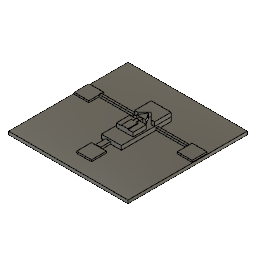
fixture v5 (Autodesk Fusion 360 design; units mm, degrees)
Autodesk Fusion 360 part; units mm, degrees
sketch "base plate" plane through (0, 0, 0) normal (0, 0, 1) x (1, 0, 0)
  line L0 (-228.6, 228.6) -> (228.6, 228.6)
  line L1 (228.6, 228.6) -> (228.6, -228.6)
  line L2 (228.6, -228.6) -> (-228.6, -228.6)
  line L3 (-228.6, -228.6) -> (-228.6, 228.6)
  line L4 (-228.6, 228.6) -> (228.6, -228.6) construction
  line L5 (228.6, 228.6) -> (-228.6, -228.6) construction
  dimension "d1" = 457.2
  dimension "d2" = 457.2
  constraint horizontal L0
  constraint perpendicular L0 L1
  constraint parallel L0 L2
  constraint parallel L1 L3
  constraint coincident L4 origin
  constraint coincident L5 origin
  measures "d1" distance of L1.end L2.end
  measures "d2" distance of L0.end L1.end
extrude "Extrude1" add sketch "base plate" along normal blind 12.7 makes body 1
sketch "cylinder components" plane through (0, 0, 12.7) normal (0, 0, 1) x (-1, 0, 0)
  line L0 (228.6, 228.6) -> (-228.6, 228.6)
  line L1 (-228.6, 228.6) -> (-228.6, -228.6)
  line L2 (-228.6, -228.6) -> (228.6, -228.6)
  line L3 (228.6, -228.6) -> (228.6, 228.6)
  line L4 (25.4, -114.3) -> (-50.8, -114.3)
  line L5 (-50.8, -114.3) -> (-50.8, 76.2)
  line L6 (-50.8, 76.2) -> (25.4, 76.2)
  line L7 (25.4, 76.2) -> (25.4, -114.3)
  line L8 (-168.91, -76.2) -> (-226.06, -76.2)
  line L9 (-226.06, -76.2) -> (-226.06, -19.05)
  line L10 (-226.06, -19.05) -> (-168.91, -19.05)
  line L11 (-168.91, -19.05) -> (-168.91, -76.2)
  line L12 (0, -254) -> (0, 228.6) construction
  line L13 (25.4, 114.3) -> (-31.75, 114.3)
  line L14 (-31.75, 114.3) -> (-31.75, 171.45)
  line L15 (-31.75, 171.45) -> (25.4, 171.45)
  line L16 (25.4, 171.45) -> (25.4, 114.3)
  line L17 (-50.8, -64.605) -> (-168.91, -64.605)
  line L18 (-168.91, -64.605) -> (-168.91, -56.223)
  line L19 (-168.91, -56.223) -> (-50.8, -56.223)
  line L20 (-50.8, -56.223) -> (-50.8, -64.605)
  line L21 (226.06, -76.2) -> (168.91, -76.2)
  line L22 (168.91, -76.2) -> (168.91, -19.05)
  line L23 (168.91, -19.05) -> (226.06, -19.05)
  line L24 (226.06, -19.05) -> (226.06, -76.2)
  line L25 (25.4, -66.1774) -> (168.91, -66.1774)
  line L26 (168.91, -66.1774) -> (168.91, -57.7954)
  line L27 (168.91, -57.7954) -> (25.4, -57.7954)
  line L28 (25.4, -57.7954) -> (25.4, -66.1774)
  line L29 (9.064, 76.2) -> (-9.97, 76.2)
  line L30 (-9.97, 76.2) -> (-9.97, 114.3)
  line L31 (-9.97, 114.3) -> (9.064, 114.3)
  line L32 (9.064, 114.3) -> (9.064, 76.2)
  dimension "d5" = 76.2
  dimension "d6" = 190.5
  dimension "d9" = 57.15
  dimension "d10" = 57.15
  dimension "d13" = 2.54
  dimension "d14" = 247.65
  dimension "d22" = 57.15
  dimension "d23" = 57.15
  dimension "d24" = 38.1
  dimension "d25" = 57.15
  dimension "d26" = 196.85
  dimension "d29" = 8.382
  dimension "d30" = 118.11
  dimension "d31" = 57.15
  dimension "d32" = 57.15
  dimension "d33" = 247.65
  dimension "d34" = 2.54
  dimension "d35" = 8.382
  constraint horizontal L4
  constraint vertical L5
  constraint horizontal L6
  constraint vertical L7
  constraint horizontal L8
  constraint vertical L9
  constraint horizontal L10
  constraint vertical L11
  constraint midpoint L0 L12.end
  constraint perpendicular L0 L12
  constraint horizontal L13
  constraint vertical L14
  constraint horizontal L15
  constraint vertical L16
  constraint horizontal L17
  constraint vertical L18
  constraint horizontal L19
  constraint vertical L20
  constraint coincident L11 L18.end
  constraint coincident L5 L17.start
  constraint horizontal L21
  constraint vertical L22
  constraint horizontal L23
  constraint vertical L24
  constraint horizontal L25
  constraint vertical L26
  constraint horizontal L27
  constraint vertical L28
  constraint coincident L22 L26.end
  constraint coincident L7 L25.start
  constraint horizontal L29
  constraint vertical L30
  constraint horizontal L31
  constraint vertical L32
  constraint coincident L13 L30.end
  constraint coincident L6 L29.start
  measures "d5" distance of L4.start L4.end
  measures "d6" distance of L4.start L6.end
  measures "d9" distance of L8.start L8.end
  measures "d10" distance of L8.start L10.end
  measures "d13" distance of L1 L9
  measures "d14" distance of L0 L9.end
  measures "d22" distance of L13.start L13.end
  measures "d23" distance of L13.start L15.end
  measures "d24" distance of L6 L13
  measures "d25" distance of L0 L15
  measures "d26" distance of L1 L14
  measures "d29" distance of L17 L19
  measures "d30" distance of L17.start L17.end
  measures "d31" distance of L21.start L21.end
  measures "d32" distance of L21.start L23.end
  measures "d33" distance of L0 L23
  measures "d34" distance of L3 L24
  measures "d35" distance of L25 L27
extrude "Extrude3" add sketch "cylinder components" along normal blind 15.24 contours L4 L5 L6 L7 L20 L28 L29 bodies 1
sketch "clip retention" plane through (0, 0, 27.94) normal (0, 0, 1) x (-1, 0, 0)
  line L0 (25.4, -114.3) -> (25.4, 76.2)
  line L1 (25.4, 76.2) -> (-50.8, 76.2)
  line L2 (-50.8, 76.2) -> (-50.8, -114.3)
  line L3 (-50.8, -114.3) -> (25.4, -114.3)
  line L4 (25.4, -50.8) -> (12.7, -50.8)
  line L5 (12.7, -50.8) -> (-12.7, -76.2)
  line L6 (-12.7, -76.2) -> (-38.1, -50.8)
  line L7 (-38.1, -50.8) -> (-50.8, -50.8)
  line L8 (-50.8, -114.3) -> (25.4, -114.3)
  line L9 (25.4, -50.8) -> (25.4, -114.3)
  line L10 (19.05, -25.4) -> (-44.45, -25.4)
  line L11 (-44.45, -25.4) -> (-44.45, 25.4)
  line L12 (-44.45, 25.4) -> (19.05, 25.4)
  line L13 (19.05, 25.4) -> (19.05, -25.4)
  line L14 (-50.8, -50.8) -> (-50.8, -52.9164)
  line L15 (-50.8, -50.8) -> (-50.8, -114.3)
  point P0 (-12.7, -76.2)
  point P1 (-50.8, -114.3)
  point P2 (25.4, -114.3)
  dimension "d41" = 50.8
  dimension "d42" = 6.35
  dimension "d43" = 6.35
  dimension "d44" = 50.8
  constraint coincident L0 L4.start
  constraint coincident P0 L5.end
  constraint perpendicular L5 L6
  constraint parallel L4 L7
  constraint coincident P1 L2.end
  constraint horizontal L10
  constraint vertical L11
  constraint horizontal L12
  constraint vertical L13
  constraint coincident L2 L14.end
  constraint perpendicular L8 L9
  constraint perpendicular L8 L15
  measures "d41" distance of L10.end L11.end
  measures "d42" distance of L2 L11
  measures "d43" distance of L0 L13
  measures "d44" distance of L1 L12
extrude "Extrude4" add sketch "cylinder components" along normal blind 6.35 contours L21 L22 L23 L24 L26 | L8 L9 L10 L11 L18 | L13 L14 L15 L16 L31 bodies 1
extrude "Extrude5" add sketch "cylinder components" along normal blind 8.382 contours L7 L22 L25 L26 L27 L28 | L5 L11 L17 L18 L19 L20 | L6 L13 L29 L30 L31 L32 bodies 1
extrude "Extrude6" add sketch "clip retention" along normal blind 15.24 contours L0 L2 L3 L4 L5 L6 L7 L8 L9 L14 L15 | L10 L11 L12 L13 bodies 1
sketch "clip hammer post cut out" plane through (0, 0, 43.18) normal (0, 0, 1) x (-1, 0, 0)
  line L0 (19.05, 25.4) -> (-44.45, 25.4)
  line L1 (-44.45, 25.4) -> (-44.45, -25.4)
  line L2 (-44.45, -25.4) -> (19.05, -25.4)
  line L3 (19.05, -25.4) -> (19.05, 25.4)
  line L4 (0, -12.7) -> (-25.4, -12.7)
  line L5 (-25.4, -12.7) -> (-25.4, 25.4)
  line L6 (-25.4, 25.4) -> (0, 25.4)
  line L7 (0, 25.4) -> (0, -12.7)
  line L8 (-7.2894, -38.3626) -> (-18.4141, -38.3626)
  line L9 (-18.4141, -38.3626) -> (-18.4141, -12.7)
  line L10 (-18.4141, -12.7) -> (-7.2894, -12.7)
  line L11 (-7.2894, -12.7) -> (-7.2894, -38.3626)
  dimension "d47" = 38.1
  constraint horizontal L4
  constraint vertical L5
  constraint horizontal L6
  constraint vertical L7
  constraint horizontal L8
  constraint vertical L9
  constraint horizontal L10
  constraint vertical L11
  constraint coincident L4 L9.end
  measures "d47" distance of L4.end L5.end
extrude "Extrude7" cut sketch "clip hammer post cut out" against normal blind 12.7 contours L0 L4 L5 L6 L7 L10 | L2 L8 L9 L11 | L2 L4 L9 L10 L11 bodies 1
sketch "clip hammer post" plane through (0, 0, 30.48) normal (0, 0, 1) x (-1, 0, 0)
  line L0 (-18.4141, -25.4) -> (-7.2894, -25.4)
  line L1 (-7.2894, -25.4) -> (-7.2894, -12.7)
  line L2 (-7.2894, -12.7) -> (0, -12.7)
  line L3 (0, -12.7) -> (0, 25.4)
  line L4 (0, 25.4) -> (-25.4, 25.4)
  line L5 (-25.4, 25.4) -> (-25.4, -12.7)
  line L6 (-25.4, -12.7) -> (-18.4141, -12.7)
  line L7 (-18.4141, -12.7) -> (-18.4141, -25.4)
  line L8 (-7.2894, -25.4) -> (-7.2894, -12.7)
  line L9 (0, -12.7) -> (0, 25.4)
  line L10 (-25.4, 25.4) -> (-25.4, -12.7)
  line L11 (-18.4141, -12.7) -> (-18.4141, -25.4)
  line L12 (-7.2894, -25.4) -> (-18.4141, -25.4)
  line L13 (0, 25.4) -> (-25.4, 25.4)
  constraint coincident L0.end L1.start
  constraint coincident L1.end L2.start
  constraint coincident L2.end L3.start
  constraint coincident L3.end L4.start
  constraint coincident L4.end L5.start
  constraint coincident L5.end L6.start
  constraint coincident L6.end L7.start
  constraint coincident L0.start L7.end
extrude "Extrude8" add sketch "clip hammer post" along normal blind 15.24 bodies 1
sketch "clip hammer" plane through (0, 0, 30.48) normal (0, 0, 1) x (1, 0, 0)
  line L0 (-5.08, 38.1) -> (30.8356, 38.1)
  line L1 (30.8356, 38.1) -> (12.8778, 65.9493)
  line L2 (12.8778, 65.9493) -> (-5.08, 38.1)
  dimension "d54" = 35.9156
  measures "d54" distance of L0.start L0.end
extrude "Extrude9" add sketch "clip hammer" along normal blind 15.24 separate body makes body 2
sketch "Sketch7" plane through (0, 0, 27.94) normal (0, 0, 1) x (-1, 0, 0)
  line L0 (-50.8, -50.8) -> (-38.1, -50.8)
  line L1 (-38.1, -50.8) -> (-12.7, -76.2)
  line L2 (-12.7, -76.2) -> (12.7, -50.8)
  line L3 (12.7, -50.8) -> (25.4, -50.8)
  line L4 (25.4, -50.8) -> (25.4, 76.2)
  line L5 (25.4, 76.2) -> (-50.8, 76.2)
  line L6 (-50.8, 76.2) -> (-50.8, -50.8)
  line L7 (19.05, 25.4) -> (19.05, -25.4)
  line L8 (19.05, -25.4) -> (-44.45, -25.4)
  line L9 (-44.45, -25.4) -> (-44.45, 25.4)
  line L10 (-44.45, 25.4) -> (19.05, 25.4)
  line L11 (-6.5765, -38.1) -> (-18.4141, -38.1)
  line L12 (-18.4141, -38.1) -> (-18.4141, -25.4)
  line L13 (-18.4141, -25.4) -> (-6.5765, -25.4)
  line L14 (-6.5765, -25.4) -> (-6.5765, -38.1)
  line L15 (5.08, -38.1) -> (-30.8356, -38.1)
  point P0 (-18.4141, -25.4)
  constraint horizontal L11
  constraint vertical L12
  constraint horizontal L13
  constraint vertical L14
  constraint coincident P0 L12.end
  constraint coincident L11.start L15
extrude "Extrude10" add sketch "Sketch7" along normal blind 15.24 contours L8 L11 L12 L13 L14 L15 bodies 1 2
named bodies: "base plate"
